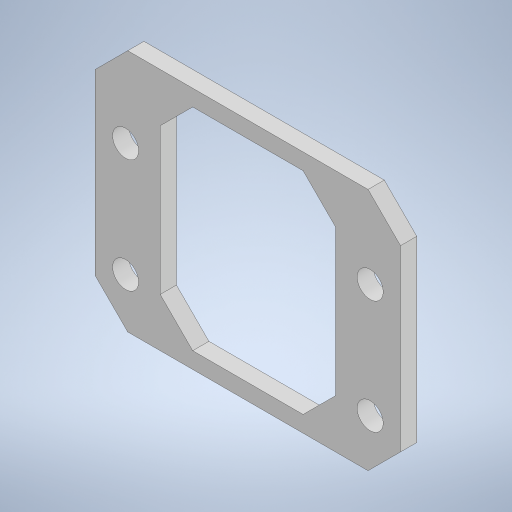
# Autodesk Inventor part: стена_простая
Saved by Autodesk Inventor 2023.1 (Build 271208000, 208)
## iProperties
Created: 2025-12-16
Part Number: стена_простая
Material: Типовые
Document SubType Name: Modeling
Designer: DELL
Density: 1 g/cm^3
Appearance: По умолчанию
Author: DELL
Autodesk Inventor part; units mm, degrees
ref_plane "YZ Plane" through (0, 0, 0) normal (1, 0, 0) x (0, 1, 0)
ref_plane "XZ Plane" through (0, 0, 0) normal (0, 1, 0) x (-1, 0, 0)
ref_plane "XY Plane" through (0, 0, 0) normal (0, 0, 1) x (1, 0, 0)
sketch "Эскиз1" plane through (0, 0, 0) normal (0, 0, 1) x (1, 0, 0)
  line L0 (-18.8, -15) -> (18.8, -15)
  line L1 (18.8, -15) -> (18.8, 15)
  line L2 (18.8, 15) -> (-18.8, 15)
  line L3 (-18.8, 15) -> (-18.8, -15)
  line L4 (-18.8, -15) -> (18.8, 15) construction
  line L5 (18.8, -15) -> (-18.8, 15) construction
  line L6 (10.8, 13) -> (-10.8, 13)
  line L7 (-10.8, 13) -> (-10.8, -13)
  line L8 (-10.8, -13) -> (10.8, -13)
  line L9 (10.8, -13) -> (10.8, 13)
  line L10 (10.8, 13) -> (-10.8, -13) construction
  line L11 (-10.8, 13) -> (10.8, -13) construction
  circle A0 centre (-15.061, 5) radius 1.6
  circle A1 centre (-15.061, -9) radius 1.6
  line L12 (0, 0) -> (0, -15) construction
  circle A2 centre (15.061, 5) radius 1.6
  circle A3 centre (15.061, -9) radius 1.6
  dimension "d0" = 37.6
  dimension "d1" = 30
  dimension "d2" = 8
  dimension "d3" = 2
  dimension "d4" = 3.2
  dimension "d5" = 3.2
  dimension "d6" = 10
  dimension "d7" = 14
  constraints: 26 end point, 5 midpoint, 4 centre point, 4 parallel, 2 horizontal, 2 perpendicular, 2 symmetric about line, 2 other
  measures "d0" distance of L2.end L1.end
  measures "d1" distance of L1.end L0.end
  measures "d2" distance between parallel lines of L3 L7
  measures "d3" distance between parallel lines of L2 L6
  measures "d4" diameter of A0
  measures "d5" diameter of A1
  measures "d6" distance from line of L2 A0.centre
  measures "d7" distance of A1.centre A0.centre
extrude "Выдавливание1" add sketch "Эскиз1" along normal blind 2
chamfer "Фаска1" distance 4 angle 45 4 edges at (18.8, 15, 1) (-18.8, 15, 1) (18.8, -15, 1) (-18.8, -15, 1)
chamfer "Фаска2" distance 4 angle 45 4 edges at (-10.8, 13, 1) (10.8, 13, 1) (10.8, -13, 1) (-10.8, -13, 1)
